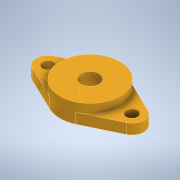
# Autodesk Inventor part: O_Do_Lan
Saved by Autodesk Inventor 2022 (Build 260153000, 153)
## iProperties
Created: 2022-11-10
Part Number: O_Do_Lan
Material: Brass, Soft Yellow, Welded
Document SubType Name: Modeling
Designer: nguye
Density: 8.5 g/cm^3
Appearance: Weld - Brass
Author: nguye
Autodesk Inventor part; units mm, degrees
ref_plane "YZ Plane" through (0, 0, 0) normal (1, 0, 0) x (0, 1, 0)
ref_plane "XZ Plane" through (0, 0, 0) normal (0, 1, 0) x (-1, 0, 0)
ref_plane "XY Plane" through (0, 0, 0) normal (0, 0, 1) x (1, 0, 0)
sketch "Sketch1" plane through (0, 0, 0) normal (0, 1, 0) x (-1, 0, 0)
  circle A0 centre (0, 0) radius 13.25
  circle A1 centre (0, 0) radius 4
  dimension "d0" = 26.5
  dimension "d1" = 8
  constraints: 2 centre point, 2 coincident
  measures "d0" diameter of A0
  measures "d1" diameter of A1
extrude "Extrusion1" add sketch "Sketch1" along normal blind 8.5
sketch "Sketch2" plane through (0, 0, 0) normal (0, -1, 0) x (1, 0, 0)
  circle A0 centre (18.5, 0) radius 2.5
  circle A1 centre (-18.5, 0) radius 2.5
  circle A2 centre (18.5, 0) radius 5.25
  circle A3 centre (-18.5, 0) radius 5.25
  line L0 (20.7703, -4.7337) -> (5.7297, -11.9471)
  circle A4 centre (0, 0) radius 13.25 projected
  line L1 (20.7703, 4.7337) -> (5.7297, 11.9471)
  line L2 (-5.7297, -11.9471) -> (-20.7703, -4.7337)
  line L3 (-5.7297, 11.9471) -> (-20.7703, 4.7337)
  point P0 (0, 18.5)
  point P1 (0, -18.5)
  dimension "d6" = 5
  dimension "d7" = 5
  dimension "d8" = 37
  dimension "d9" = 18.5
  dimension "d10" = 10.5
  dimension "d11" = 10.5
  dimension "d14" = 47.5
  constraints: 8 end point, 8 point on circle, 8 tangent, 4 centre point, 2 coincident, 2 horizontal alignment, 1 vertical alignment
  measures "d6" diameter of A0
  measures "d7" diameter of A1
  measures "d8" distance of A1.centre A0.centre
  measures "d9" distance of point (0, 0) A0.centre
  measures "d10" diameter of A2
  measures "d11" diameter of A3
extrude "Extrusion2" add sketch "Sketch2" against normal blind 4.5 contours A2 | A2 A4 L1 | L0 A4 A2 | A4 A3 L3 | L2 A3 A4 | A3
body "Solid1"
